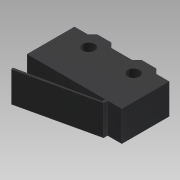
# Autodesk Inventor part: Part21
Saved by Autodesk Inventor 2014 (Build 180170000, 170)
## iProperties
Created: 2016-03-28
Part Number: Part21
Material: ABS Plastic
Document SubType Name: Modeling
Designer: admin
Density: 1.06 g/cm^3
Appearance: Dark Gray
Author: admin
Autodesk Inventor part; units mm, degrees
ref_plane "YZ Plane" through (0, 0, 0) normal (1, 0, 0) x (0, 1, 0)
ref_plane "XZ Plane" through (0, 0, 0) normal (0, 1, 0) x (-1, 0, 0)
ref_plane "XY Plane" through (0, 0, 0) normal (0, 0, 1) x (1, 0, 0)
sketch "Sketch1" plane through (0, 0, 0) normal (0, 0, 1) x (1, 0, 0)
  line L0 (13.5, -2.5) -> (13.5, 0) projected
  line L1 (12, 0) -> (13.5, 0) projected
  line L2 (12, 0) -> (12, -2) projected
  arc A0 (8, -2) -> (12, -2) centre (10, -2) ccw projected
  line L3 (8, -2) -> (8, 0) projected
  line L4 (6.5, 0) -> (8, 0) projected
  line L5 (6.5, 0) -> (6.5, -2.5) projected
  line L6 (6.5, -2.5) -> (4, -2.5) projected
  line L7 (4, -2.5) -> (4, 0) projected
  line L8 (0, 0) -> (4, 0) projected
  line L9 (0, 0) -> (0, -8) projected
  line L10 (20, -8) -> (0, -8) projected
  line L11 (20, 0) -> (20, -8) projected
  line L12 (16, 0) -> (20, 0) projected
  line L13 (16, 0) -> (16, -2.5) projected
  line L14 (16, -2.5) -> (13.5, -2.5) projected
  circle A1 centre (5.25, -1.25) radius 1.25
  circle A2 centre (14.75, -1.25) radius 1.25
  line L15 (20, 1) -> (20, -9)
  line L16 (20, -9) -> (0, -9)
  line L17 (0, -9) -> (0, 1)
  line L18 (0, 1) -> (20, 1)
  line L19 (17.25, 1) -> (16.25, 2)
  line L20 (13.25, 2) -> (12.25, 1)
  line L21 (7.75, 1) -> (6.75, 2)
  line L22 (2.75, 1) -> (3.75, 2)
  line L23 (3.75, 2) -> (6.75, 2)
  line L24 (13.25, 2) -> (16.25, 2)
  dimension "d0" = 9
  dimension "d3" = 45
  dimension "d4" = 45
  dimension "d5" = 45
  dimension "d6" = 3
  dimension "d7" = 3
  dimension "d8" = 1.5
  dimension "d9" = 2.5
  dimension "d10" = 2.5
  dimension "d11" = 1.5
  constraints: 20 end point, 4 parallel, 4 point on line, 3 perpendicular, 2 centre point, 2 horizontal, 2 tangent
  measures "d0" distance between parallel lines of L12 L16
  measures "d3" angle of L18 L22
  measures "d4" angle of L18 L21
  measures "d5" angle of L18 L19
  measures "d6" distance of L22.end L21.end
  measures "d7" distance of L19.end L20.start
  measures "d8" horizontal distance of L22.end A1.centre
  measures "d9" diameter of A1
  measures "d10" diameter of A2
  measures "d11" horizontal distance of L19.end A2.centre
extrude "Extrusion1" add sketch "Sketch1" along normal blind 6.4 contours L14 L13 L12 L11 L10 L9 L8 L7 L6 L5 L4 L3 A0 L2 L1 L0 | L0 A2 L14 | L0 L1 L2 A0 L3 L4 L5 A1 L7 L8 L17 L18 L15 L12 L13 A2 | A2 L13 L14 | L15 L16 L17 L10 | L18 L20 L24 L19 | L5 L6 A1 | L18 L22 L23 L21 | A1 L6 L7
sketch "Sketch2" plane through (0, 0, 6.4) normal (0, 0, 1) x (1, 0, 0)
  line L0 (0, -9) -> (20, -9) projected
  line L1 (20, 1) -> (17.25, 1) projected
  line L2 (16.5219, -9) -> (16.5219, -9.7169)
  line L3 (16.5219, -9.7169) -> (1, -13)
  line L4 (1, -13) -> (1.0938, -13.4435)
  line L5 (1.0938, -13.4435) -> (17, -9.8474)
  line L6 (17, -9.8474) -> (17, -9)
  point P0 (0, 0)
  constraints: 10 end point, 2 perpendicular, 2 point on line, 1 parallel
extrude "Extrusion2" add sketch "Sketch2" against normal blind 6.4
body "Solid1"
